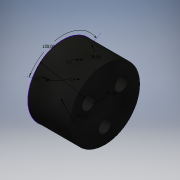
# Autodesk Inventor part: каркас
Saved by Autodesk Inventor 2019 (Build 230136000, 136)
## iProperties
Created: 2019-07-16
Part Number: каркас
Material: Пластмасса, непрозрачная, черная
Document SubType Name: Modeling
Designer: Boss
Mass: 0.429194 g
Surface Area: 3.95715 cm^2
Volume: 0.450834 cm^3
Density: 0.952 g/cm^3
Appearance: Гладкая — черная
Author: Boss
Autodesk Inventor part; units mm, degrees
ref_plane "YZ Plane" through (0, 0, 0) normal (1, 0, 0) x (0, 1, 0)
ref_plane "XZ Plane" through (0, 0, 0) normal (0, 1, 0) x (-1, 0, 0)
ref_plane "XY Plane" through (0, 0, 0) normal (0, 0, 1) x (1, 0, 0)
sketch "Эскиз1" plane through (0, 0, 0) normal (1, 0, 0) x (0, 1, 0)
  circle A0 centre (0, 0) radius 5
  circle A1 centre (0, -2.7) radius 0.6
  circle A2 centre (0, 0) radius 2.7 construction
  circle A3 centre (-2.3383, 1.35) radius 0.6
  circle A4 centre (2.3383, 1.35) radius 0.6
  line L0 (0, 0) -> (5.4782, 3.1628) construction
  line L1 (0, 0) -> (-5.2011, 3.0029) construction
  line L2 (0, 0) -> (5.5612, 0) construction
  point P0 (2.3383, 1.35)
  dimension "d1" = 10
  dimension "d3" = 1.2
  dimension "d24" = 5.4
  dimension "d25" = 1.2
  dimension "d26" = 1.2
  dimension "d53" = 120
  dimension "d54" = 30
  constraints: 6 end point, 5 centre point, 5 coincident, 3 point on circle, 2 point on line, 1 horizontal, 1 vertical alignment
  measures "d1" diameter of A0
  measures "d3" diameter of A1
  measures "d24" diameter of A2
  measures "d25" diameter of A3
  measures "d26" diameter of A4
  measures "d53" angle of L1 L0
  measures "d54" angle of L2 L0
extrude "Выдавливание1" add sketch "Эскиз1" along normal blind 6 contours A0 | A3 | A4
sketch "Эскиз4" plane through (6, 0, 0) normal (1, 0, 0) x (0, 0, -1)
  circle A0 centre (2.7, 0) radius 0.6 projected
  point P0 (-1.35, 2.3383)
  point P1 (-1.35, 2.3383)
  constraints: 1 coincident
hole "Отверстие2" at (6, 0, -2.7) direction (-1, 0, 0) diameter 1.7 depth 3
extrude "Выдавливание2" cut sketch "Эскиз1" along normal blind 6 contours A3 | A4
sketch "Эскиз2" plane through (6, 0, 0) normal (1, 0, 0) x (0, 0, -1)
  point P0 (0, 0)
  point P1 (-1.35, 2.3383)
  point P2 (-1.35, 2.3383)
  constraints: 1 coincident
hole "Отверстие4" at (6, 2.3383, 1.35) direction (-1, 0, 0) diameter 1.8 depth 3
sketch "Эскиз3" plane through (6, 0, 0) normal (1, 0, 0) x (0, 0, -1)
  point P0 (0, 0)
  point P1 (-1.35, -2.3383)
  point P2 (-1.35, -2.3383)
  constraints: 1 coincident
hole "Отверстие5" at (6, -2.3383, 1.35) direction (-1, 0, 0) diameter 1.8 depth 3
equation "\"d1\" = inside"
equation "\"d3\" = 2 * pin_small_rad"
equation "\"d17\" = pin_big_dia"
equation "\"inside\" = 10"
equation "\"pin_small_rad\" = 0.6"
equation "\"pin_big_dia\" = 1.7"
